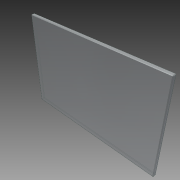
# Autodesk Inventor part: controller_lcd_cover_glass
Saved by Autodesk Inventor 2014 (Build 180170000, 170)
## iProperties
Created: 2014-03-22
Part Number: controller_lcd_cover_glass
Material: Glass
Document SubType Name: Modeling
Designer: buben
Density: 2.18 g/cm^3
Appearance: Clear
Author: buben
Autodesk Inventor part; units mm, degrees
ref_plane "YZ Plane" through (0, 0, 0) normal (1, 0, 0) x (0, 1, 0)
ref_plane "XZ Plane" through (0, 0, 0) normal (0, 1, 0) x (-1, 0, 0)
ref_plane "XY Plane" through (0, 0, 0) normal (0, 0, 1) x (1, 0, 0)
sketch "Sketch1" plane through (0, 0, 0) normal (0, 1, 0) x (-1, 0, 0)
  line L0 (0, 0) -> (-78.5, 0)
  line L1 (-78.5, 0) -> (-78.5, -51.5)
  line L2 (-78.5, -51.5) -> (0, -51.5)
  line L3 (0, -51.5) -> (0, 0)
  dimension "d0" = 78.5
  dimension "d1" = 51.5
  constraints: 8 end point, 2 parallel, 1 horizontal, 1 perpendicular
  measures "d0" distance of L0.start L0.end
  measures "d1" distance of L2.end L0.start
extrude "Extrusion1" add sketch "Sketch1" along normal blind 2
chamfer "Chamfer1" distance 0.3 angle 45 12 edges at (0, 2, -25.75) (39.25, 2, 0) (39.25, 2, -51.5) (78.5, 2, -25.75) (78.5, 0, -25.75) (39.25, 0, 0) (0, 0, -25.75) (39.25, 0, -51.5) (0, 1, -51.5) (0, 1, 0) (78.5, 1, -51.5) (78.5, 1, 0)
body "Solid1"
